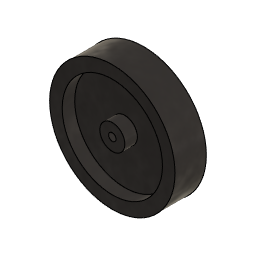
Wheel v3 (Autodesk Fusion 360 design; units mm, degrees)
Autodesk Fusion 360 part; units mm, degrees
sketch "Sketch1" plane through (0, 0, 0) normal (0, 1, 0) x (1, 0, 0)
  circle A0 centre (0, 0) radius 50
  dimension "d1" = 100
  constraint coincident A0.centre origin
  measures "d1" diameter of A0
extrude "Extrude1" add sketch "Sketch1" along normal mid plane 25
sketch "Sketch2" plane through (0, -12.5, 0) normal (0, -1, 0) x (1, 0, 0)
  circle A0 centre (0, 0) radius 50
  circle A1 centre (0, 0) radius 40
  dimension "d4" = 80
  constraint coincident A0.centre A1.centre
  measures "d4" diameter of A1
extrude "Extrude2" cut sketch "Sketch2" against normal blind 10 contours A1
sketch "Sketch3" plane through (0, 12.5, 0) normal (0, 1, 0) x (-1, 0, 0)
  circle A0 centre (0, 0) radius 50
  circle A1 centre (0, 0) radius 40
  dimension "d7" = 80
  constraint coincident A0.centre A1.centre
  measures "d7" diameter of A1
extrude "Extrude3" cut sketch "Sketch3" against normal blind 10 contours A1
sketch "Sketch4" plane through (0, -2.5, 0) normal (0, -1, 0) x (1, 0, 0)
  circle A0 centre (0, 0) radius 40
  circle A1 centre (0, 0) radius 10
  dimension "d10" = 20
  constraint coincident A0.centre A1.centre
  measures "d10" diameter of A1
extrude "Extrude4" add sketch "Sketch4" along normal blind 10 contours A1
sketch "Sketch5" plane through (0, 2.5, 0) normal (0, 1, 0) x (-1, 0, 0)
  circle A0 centre (0, 0) radius 40
  circle A1 centre (0, 0) radius 10
  dimension "d13" = 20
  constraint coincident A0.centre A1.centre
  measures "d13" diameter of A1
extrude "Extrude5" add sketch "Sketch5" along normal blind 10 contours A1
sketch "Sketch6" plane through (0, 12.5, 0) normal (0, 1, 0) x (-1, 0, 0)
  circle A0 centre (0, 0) radius 10
  circle A1 centre (0, 0) radius 3
  dimension "d16" = 6
  constraint coincident A0.centre A1.centre
  measures "d16" diameter of A1
extrude "Extrude6" cut sketch "Sketch6" against normal blind 25 contours A1
